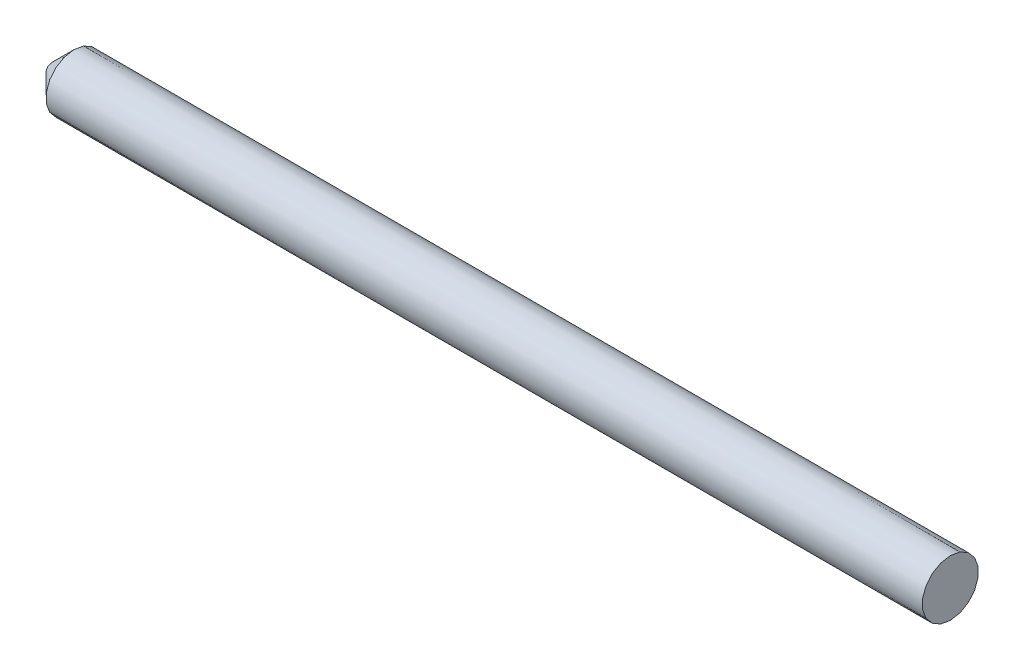
# Autodesk Inventor part: Shaft
Saved by Autodesk Inventor 2016 (Build 200138000, 138)
## iProperties
Created: 2015-10-31
Part Number: Shaft
Material: Steel
Document SubType Name: Modeling
Designer: rossmosier
Density: 1 g/cm^3
Appearance: Steel
CustomPartVersion: 1
d0: 0.000 in
d1: 0.000 in
d2: 0.00 deg
Author: rossmosier
Autodesk Inventor part; units mm, degrees
ref_plane "Start Plane" through (0, 0, 0) normal (1, 0, 0) x (0, 1, 0)
ref_plane "XZ Plane" through (0, 0, 0) normal (0, 1, 0) x (-1, 0, 0)
ref_plane "XY Plane" through (0, 0, 0) normal (0, 0, 1) x (1, 0, 0)
sketch "Main Sketch" plane through (0, 0, 0) normal (0, 0, 1) x (1, 0, 0)
  line L0 (0, 0) -> (101.6, 0)
  line L1 (0, 0) -> (0, 3.175)
  line L2 (101.6, 3.175) -> (101.6, 0)
  line L3 (0, 3.175) -> (101.6, 3.175)
  dimension "d3" = 6.35
  constraints: 8 end point, 2 vertical, 1 horizontal
  measures "d3" diameter of L3 L0
revolve "Revolution1" add sketch "Main Sketch" angle 360 about axis through (0, 0, 0) along (1, 0, 0)
chamfer "Chamfer2" distance 2.54 angle 45 1 edges at (0, -3.175, 0) measured on face at (0.5, -3.175, 0)
body "Solid1"
